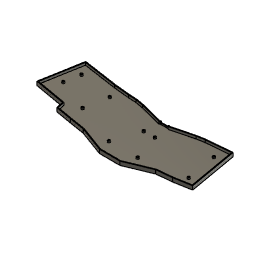
quetzal - minimal - lowpro (Autodesk Fusion 360 design; units mm, degrees)
Autodesk Fusion 360 part; units mm, degrees
note: some values were not read from the file. Set by a fixed rule: which sketch regions a step uses.
(part 1 of 15)
sketch "atreuskeypad-Edge_Cuts" plane through (0, 0, 0) normal (0, 1, 0) x (1, 0, 0)
  line L0 (156.651, -54.9359) -> (156.645, -54.9431)
  line L1 (156.607, -54.9484) -> (101.099, -40.5089)
  line L2 (25.155, -32.2997) -> (25.1539, -32.2991)
  line L3 (156.645, -54.9431) -> (156.635, -54.9446)
  line L4 (63.165, -36.1397) -> (25.155, -32.2997)
  line L5 (177.784, -54.9772) -> (177.776, -54.9799)
  line L6 (176.132, -52.9608) -> (176.134, -52.9601)
  line L7 (329.099, -144.851) -> (329.095, -144.87)
  line L8 (176.165, -52.9746) -> (176.166, -52.9765)
  line L9 (329.091, -144.889) -> (329.091, -144.889)
  line L10 (156.602, -54.8436) -> (158.121, -52.9883)
  line L11 (158.14, -52.9782) -> (158.155, -52.9702)
  line L12 (309.232, -32.2617) -> (309.24, -32.2769)
  line L13 (329.091, -144.889) -> (329.076, -144.898)
  line L14 (252.021, -37.1608) -> (252.024, -37.1613)
  line L15 (309.23, -32.261) -> (309.232, -32.2617)
  line L16 (63.1661, -36.1394) -> (63.165, -36.1397)
  line L17 (158.158, -52.971) -> (158.16, -52.97)
  line L18 (82.3387, -37.1108) -> (101.119, -40.4108)
  line L19 (177.766, -54.9747) -> (177.755, -54.9731)
  line L20 (25.1526, -32.2995) -> (-56.8492, -20.0866)
  line L21 (63.1672, -36.1399) -> (63.1661, -36.1394)
  line L22 (158.121, -52.9883) -> (158.124, -52.9871)
  line L23 (25.1539, -32.2991) -> (25.1526, -32.2995)
  line L24 (158.155, -52.9702) -> (158.158, -52.971)
  line L25 (329.091, -144.889) -> (329.091, -144.889)
  line L26 (309.212, -32.2553) -> (309.229, -32.259)
  line L27 (309.249, -32.2913) -> (329.099, -144.851)
  line L28 (233.247, -40.4916) -> (233.25, -40.4919)
  line L29 (329.099, -144.851) -> (329.099, -144.851)
  line L30 (158.124, -52.9871) -> (158.125, -52.9847)
  line L31 (176.168, -52.9774) -> (177.798, -54.8738)
  line L32 (177.798, -54.8738) -> (233.247, -40.4916)
  line L33 (-73.4847, -113.859) -> (-73.501, -113.849)
  line L34 (309.196, -32.2502) -> (309.212, -32.2553)
  line L35 (63.1739, -36.0401) -> (82.3328, -37.1101)
  line L36 (309.24, -32.2769) -> (309.249, -32.2913)
  line L37 (176.107, -53.06) -> (158.184, -53.07)
  line L38 (158.16, -52.97) -> (176.13, -52.96)
  line L39 (101.099, -40.5089) -> (82.3243, -37.2098)
  line L40 (177.755, -54.9731) -> (177.75, -54.9664)
  line L41 (329.095, -144.87) -> (329.091, -144.889)
  line L42 (158.184, -53.07) -> (156.659, -54.9317)
  line L43 (156.625, -54.9498) -> (156.616, -54.9471)
  line L44 (82.3356, -37.1114) -> (82.3387, -37.1108)
  line L45 (177.793, -54.9784) -> (177.784, -54.9772)
  line L46 (176.149, -52.968) -> (176.165, -52.9746)
  line L47 (252.024, -37.1613) -> (252.026, -37.1602)
  line L48 (233.25, -40.4919) -> (233.251, -40.4908)
  line L49 (82.3328, -37.1101) -> (82.3356, -37.1114)
  line L50 (156.659, -54.9317) -> (156.651, -54.9359)
  line L51 (156.616, -54.9471) -> (156.607, -54.9484)
  line L52 (176.134, -52.9601) -> (176.149, -52.968)
  line L53 (177.742, -54.9626) -> (176.107, -53.06)
  line L54 (177.75, -54.9664) -> (177.742, -54.9626)
  line L55 (176.166, -52.9765) -> (176.168, -52.9774)
  line L56 (82.3243, -37.2098) -> (63.1672, -36.1399)
  line L57 (177.776, -54.9799) -> (177.766, -54.9747)
  line L58 (-56.8492, -20.0866) -> (-73.4021, -113.779)
  line L59 (156.635, -54.9446) -> (156.625, -54.9498)
  line L60 (101.12, -40.4119) -> (101.123, -40.4116)
  line L61 (176.13, -52.96) -> (176.132, -52.9608)
  line L62 (101.119, -40.4108) -> (101.12, -40.4119)
  line L63 (233.251, -40.4908) -> (252.021, -37.1608)
  line L64 (158.125, -52.9847) -> (158.14, -52.9782)
  line L65 (25.1662, -32.2004) -> (63.1739, -36.0401)
  line L66 (101.123, -40.4116) -> (156.602, -54.8436)
  line L67 (309.229, -32.259) -> (309.23, -32.261)
  line L68 (252.026, -37.1602) -> (309.196, -32.2502)
  line L69 (329.099, -144.851) -> (329.099, -144.851)
  line L70 (191.739, -180.826) -> (191.729, -180.826)
  line L71 (-73.501, -113.849) -> (-73.501, -113.849)
  line L72 (5.3213, -144.859) -> (5.3127, -144.854)
  line L73 (80.4872, -157.589) -> (42.832, -151.479)
  line L74 (142.913, -180.577) -> (80.4872, -157.589)
  line L75 (291.525, -151.51) -> (253.532, -155.399)
  line L76 (5.3027, -144.852) -> (5.2973, -144.844)
  line L77 (-56.9191, -19.9896) -> (-56.9187, -19.989)
  line L78 (1.611, -127.061) -> (1.6132, -127.071)
  line L79 (-56.9293, -20.0057) -> (-56.9198, -19.9898)
  line L80 (1.5787, -127.041) -> (1.5873, -127.046)
  line L81 (-73.5092, -113.811) -> (-73.5092, -113.811)
  line L82 (5.3127, -144.854) -> (5.3027, -144.852)
  line L83 (5.2868, -144.829) -> (5.2811, -144.82)
  line L84 (-56.9006, -19.985) -> (-56.8826, -19.9805)
  line L85 (291.513, -151.41) -> (328.992, -144.819)
  line L86 (-56.9198, -19.9898) -> (-56.9191, -19.9896)
  line L87 (253.501, -155.304) -> (253.508, -155.304)
  line L88 (253.532, -155.399) -> (191.739, -180.826)
  line L89 (-73.5054, -113.829) -> (-73.5092, -113.811)
  line L90 (5.2973, -144.844) -> (5.289, -144.839)
  line L91 (1.5281, -127.133) -> (-73.4687, -113.869)
  line L92 (142.93, -180.58) -> (142.922, -180.577)
  line L93 (80.5123, -157.493) -> (80.5173, -157.493)
  line L94 (-73.4021, -113.779) -> (1.5787, -127.041)
  line L95 (-56.9392, -20.0213) -> (-56.9293, -20.0057)
  line L96 (1.5973, -127.048) -> (1.6028, -127.056)
  line L97 (329.059, -144.909) -> (291.529, -151.509)
  line L98 (328.992, -144.819) -> (309.159, -32.3537)
  line L99 (-73.5092, -113.811) -> (-73.5092, -113.811)
  line L100 (329.076, -144.898) -> (329.059, -144.909)
  line L101 (42.8317, -151.479) -> (42.8313, -151.479)
  line L102 (1.6028, -127.056) -> (1.611, -127.061)
  line L103 (-56.8826, -19.9805) -> (25.1662, -32.2004)
  line L104 (80.5173, -157.493) -> (142.939, -180.48)
  line L105 (191.71, -180.73) -> (253.501, -155.304)
  line L106 (291.527, -151.509) -> (291.525, -151.51)
  line L107 (5.3719, -144.767) -> (42.8483, -151.381)
  line L108 (1.6132, -127.071) -> (1.6189, -127.08)
  line L109 (142.939, -180.48) -> (191.71, -180.73)
  line L110 (1.6189, -127.08) -> (5.3719, -144.767)
  line L111 (253.508, -155.304) -> (253.515, -155.3)
  line L112 (-73.5092, -113.811) -> (-73.5092, -113.811)
  line L113 (5.2811, -144.82) -> (1.5281, -127.133)
  line L114 (5.289, -144.839) -> (5.2868, -144.829)
  line L115 (42.8483, -151.381) -> (80.508, -157.491)
  line L116 (1.5873, -127.046) -> (1.5973, -127.048)
  line L117 (-73.5092, -113.811) -> (-56.9392, -20.0213)
  line L118 (80.508, -157.491) -> (80.5123, -157.493)
  line L119 (253.515, -155.3) -> (291.513, -151.41)
  line L120 (42.832, -151.479) -> (42.8317, -151.479)
  line L121 (142.922, -180.577) -> (142.913, -180.577)
  line L122 (-73.501, -113.849) -> (-73.5054, -113.829)
  line L123 (-56.9187, -19.989) -> (-56.9006, -19.985)
  line L124 (233.271, -40.5889) -> (177.793, -54.9784)
  line L125 (329.059, -144.909) -> (329.059, -144.909)
  line L126 (191.72, -180.83) -> (142.93, -180.58)
  line L127 (42.8313, -151.479) -> (5.3213, -144.859)
  line L128 (191.729, -180.826) -> (191.72, -180.83)
  line L129 (309.159, -32.3537) -> (252.037, -37.2596)
  line L130 (-73.501, -113.849) -> (-73.501, -113.849)
  line L131 (291.529, -151.509) -> (291.527, -151.509)
  line L132 (-73.4687, -113.869) -> (-73.4847, -113.859)
  line L133 (329.059, -144.909) -> (329.059, -144.909)
  line L134 (252.037, -37.2596) -> (233.271, -40.5889)
sketch "Sketch2" plane through (0, 0, 0) normal (0, 1, 0) x (1, 0, 0)
extrude "Extrude1" add sketch "atreuskeypad-Edge_Cuts" along normal blind 3 contours L0 L1 L3 L4 L5 L19 L20 L21 L23 L37 L39 L40 L42 L43 L45 L50 L51 L53 L54 L56 L57 L58 L59 L78 L80 L85 L87 L93 L94 L96 L98 L102 L104 L105 L107 L108 L109 L110 L111 L115 L116 L118 L119 L124 L129 L134
sketch "atreuskeypad-F_Mask" plane through (0, 0, 0) normal (0, 1, 0) x (1, 0, 0)
  line L0 (199.475, -99.2993) -> (199.496, -99.1151)
  line L1 (132.979, -99.2592) -> (133, -99.075)
  line L2 (200.247, -98.3794) -> (200.432, -98.3626)
  line L3 (316.576, -97.7949) -> (316.753, -97.8497)
  line L4 (55.7718, -103.478) -> (55.5955, -103.42)
  line L5 (297.244, -102.904) -> (297.082, -102.814)
  line L6 (37.6083, -101.631) -> (37.6619, -101.809)
  line L7 (298.401, -102.581) -> (298.28, -102.721)
  line L8 (297.605, -102.983) -> (297.42, -102.961)
  line L9 (298.492, -102.42) -> (298.401, -102.581)
  line L10 (56.1408, -103.485) -> (55.9559, -103.5)
  line L11 (55.6199, -101.669) -> (55.7978, -101.617)
  line L12 (296.751, -101.659) -> (296.841, -101.497)
  line L13 (297.082, -102.814) -> (296.941, -102.693)
  line L14 (297.968, -102.919) -> (297.789, -102.969)
  line L15 (296.69, -102.205) -> (296.675, -102.02)
  line L16 (296.675, -102.02) -> (296.695, -101.836)
  line L17 (37.2613, -101.206) -> (37.4041, -101.324)
  line L18 (296.96, -101.355) -> (297.104, -101.239)
  line L19 (287.81, -102.867) -> (287.987, -102.922)
  line L20 (40.0114, -103.894) -> (39.8851, -103.641)
  line L21 (288.15, -103.01) -> (288.293, -103.128)
  line L22 (43.6913, -103.281) -> (43.6146, -103.553)
  line L23 (40.3638, -104.333) -> (40.172, -104.126)
  line L24 (39.9368, -101.996) -> (40.0787, -101.751)
  line L25 (288.497, -103.436) -> (288.551, -103.613)
  line L26 (39.8851, -103.641) -> (39.7957, -103.373)
  line L27 (40.0787, -101.751) -> (40.2536, -101.529)
  line L28 (288.293, -103.128) -> (288.41, -103.272)
  line L29 (39.7449, -103.095) -> (39.7338, -102.813)
  line L30 (43.1691, -104.267) -> (42.9587, -104.456)
  line L31 (41.2051, -100.946) -> (41.4822, -100.891)
  line L32 (43.3509, -104.051) -> (43.1691, -104.267)
  line L33 (42.4691, -104.735) -> (42.1997, -104.82)
  line L34 (288.487, -104.184) -> (288.395, -104.345)
  line L35 (40.9386, -101.04) -> (41.2051, -100.946)
  line L36 (40.5828, -104.512) -> (40.3638, -104.333)
  line L37 (39.7338, -102.813) -> (39.7626, -102.532)
  line L38 (43.6146, -103.553) -> (43.5004, -103.811)
  line L39 (43.5004, -103.811) -> (43.3509, -104.051)
  line L40 (42.1997, -104.82) -> (41.9211, -104.867)
  line L41 (42.8309, -101.204) -> (43.0555, -101.375)
  line L42 (39.8307, -102.257) -> (39.9368, -101.996)
  line L43 (41.085, -104.768) -> (40.8249, -104.658)
  line L44 (42.7238, -104.613) -> (42.4691, -104.735)
  line L45 (41.9211, -104.867) -> (41.6386, -104.873)
  line L46 (42.0457, -100.9) -> (42.3209, -100.964)
  line L47 (109.245, -73.0347) -> (109.335, -72.8722)
  line L48 (-35.0955, -72.3151) -> (-35.1722, -72.587)
  line L49 (-35.0539, -71.9095) -> (-35.0579, -72.0351)
  line L50 (-35.2311, -71.0865) -> (-35.1333, -71.3515)
  line L51 (215.619, -98.2785) -> (215.409, -98.467)
  line L52 (1.4974, -97.4895) -> (1.6419, -97.3733)
  line L53 (215.409, -98.467) -> (215.174, -98.624)
  line L54 (-35.6177, -73.3013) -> (-35.8281, -73.4898)
  line L55 (316.916, -97.9379) -> (317.059, -98.0561)
  line L56 (133.725, -100.2) -> (133.549, -100.143)
  line L57 (133.549, -100.143) -> (133.387, -100.053)
  line L58 (-35.7313, -70.4093) -> (-35.5331, -70.6106)
  line L59 (133.264, -98.5938) -> (133.409, -98.4776)
  line L60 (133.751, -98.3393) -> (133.936, -98.3225)
  line L61 (317.176, -98.1997) -> (317.263, -98.3634)
  line L62 (133.409, -98.4776) -> (133.573, -98.3917)
  line L63 (316.753, -97.8497) -> (316.916, -97.9379)
  line L64 (133.936, -98.3225) -> (134.12, -98.3419)
  line L65 (133, -99.075) -> (133.056, -98.8983)
  line L66 (1.6419, -97.3733) -> (1.8062, -97.2874)
  line L67 (2.1687, -97.2182) -> (2.3531, -97.2376)
  line L68 (-35.4359, -73.0851) -> (-35.6177, -73.3013)
  line L69 (200.432, -98.3626) -> (200.616, -98.382)
  line L70 (134.879, -99.2725) -> (134.879, -99.299)
  line L71 (134.861, -99.088) -> (134.879, -99.2725)
  line L72 (200.769, -100.198) -> (200.59, -100.248)
  line L73 (200.045, -100.183) -> (199.883, -100.093)
  line L74 (200.59, -100.248) -> (200.405, -100.262)
  line L75 (216.142, -97.2923) -> (216.065, -97.5642)
  line L76 (212.195, -97.1062) -> (212.184, -96.8239)
  line L77 (212.908, -95.3457) -> (213.138, -95.1814)
  line L78 (212.387, -96.0068) -> (212.529, -95.7625)
  line L79 (212.335, -97.6521) -> (212.246, -97.3841)
  line L80 (212.622, -98.1372) -> (212.462, -97.9048)
  line L81 (215.281, -95.2151) -> (215.506, -95.3865)
  line L82 (121.692, -95.5477) -> (121.86, -95.775)
  line L83 (122.092, -96.2887) -> (122.151, -96.5648)
  line L84 (119.524, -98.7388) -> (119.263, -98.6287)
  line L85 (213.655, -94.9576) -> (213.932, -94.9025)
  line L86 (214.215, -94.887) -> (214.496, -94.9113)
  line L87 (214.089, -98.8845) -> (213.808, -98.8513)
  line L88 (212.814, -98.3446) -> (212.622, -98.1372)
  line L89 (213.138, -95.1814) -> (213.389, -95.0512)
  line L90 (216.183, -96.8867) -> (216.179, -97.0123)
  line L91 (120.484, -94.8713) -> (120.759, -94.9351)
  line L92 (1.9841, -97.235) -> (2.1687, -97.2182)
  line L93 (215.801, -98.0623) -> (215.619, -98.2785)
  line L94 (216.006, -96.0637) -> (216.104, -96.3287)
  line L95 (213.535, -98.7789) -> (213.275, -98.6687)
  line L96 (121.789, -98.0222) -> (121.608, -98.2385)
  line L97 (215.174, -98.624) -> (214.919, -98.7463)
  line L98 (212.529, -95.7625) -> (212.704, -95.5407)
  line L99 (122.053, -97.5241) -> (121.939, -97.7825)
  line L100 (118.45, -97.8647) -> (118.324, -97.612)
  line L101 (215.506, -95.3865) -> (215.704, -95.5878)
  line L102 (118.269, -96.2286) -> (118.375, -95.9668)
  line L103 (118.375, -95.9668) -> (118.517, -95.7225)
  line L104 (212.246, -97.3841) -> (212.195, -97.1062)
  line L105 (121.269, -95.175) -> (121.494, -95.3464)
  line L106 (212.281, -96.2687) -> (212.387, -96.0068)
  line L107 (119.126, -95.1414) -> (119.377, -95.0111)
  line L108 (213.808, -98.8513) -> (213.535, -98.7789)
  line L109 (118.517, -95.7225) -> (118.692, -95.5006)
  line L110 (119.377, -95.0111) -> (119.644, -94.9175)
  line L111 (216.104, -96.3287) -> (216.163, -96.6049)
  line L112 (213.275, -98.6687) -> (213.033, -98.523)
  line L113 (121.494, -95.3464) -> (121.692, -95.5477)
  line L114 (122.171, -96.8466) -> (122.167, -96.9722)
  line L115 (214.65, -98.8314) -> (214.371, -98.8778)
  line L116 (121.86, -95.775) -> (121.994, -96.0236)
  line L117 (214.771, -94.9751) -> (215.035, -95.0771)
  line L118 (216.163, -96.6049) -> (216.183, -96.8867)
  line L119 (120.759, -94.9351) -> (121.023, -95.037)
  line L120 (214.371, -98.8778) -> (214.089, -98.8845)
  line L121 (214.919, -98.7463) -> (214.65, -98.8314)
  line L122 (213.932, -94.9025) -> (214.215, -94.887)
  line L123 (215.035, -95.0771) -> (215.281, -95.2151)
  line L124 (121.994, -96.0236) -> (122.092, -96.2887)
  line L125 (212.213, -96.5429) -> (212.281, -96.2687)
  line L126 (213.033, -98.523) -> (212.814, -98.3446)
  line L127 (212.184, -96.8239) -> (212.213, -96.5429)
  line L128 (1.3782, -97.6315) -> (1.4974, -97.4895)
  line L129 (212.462, -97.9048) -> (212.335, -97.6521)
  line L130 (122.151, -96.5648) -> (122.171, -96.8466)
  line L131 (213.389, -95.0512) -> (213.655, -94.9576)
  line L132 (212.704, -95.5407) -> (212.908, -95.3457)
  line L133 (121.023, -95.037) -> (121.269, -95.175)
  line L134 (215.951, -97.8226) -> (215.801, -98.0623)
  line L135 (109.235, -73.7586) -> (109.184, -73.5804)
  line L136 (-35.5331, -70.6106) -> (-35.3653, -70.8378)
  line L137 (109.169, -73.3957) -> (109.189, -73.2114)
  line L138 (134.879, -99.299) -> (134.856, -99.483)
  line L139 (201.202, -99.8602) -> (201.08, -100.001)
  line L140 (199.627, -99.8272) -> (199.542, -99.6623)
  line L141 (199.542, -99.6623) -> (199.491, -99.4841)
  line L142 (200.934, -100.115) -> (200.769, -100.198)
  line L143 (199.761, -98.6338) -> (199.905, -98.5176)
  line L144 (201.08, -100.001) -> (200.934, -100.115)
  line L145 (200.221, -100.24) -> (200.045, -100.183)
  line L146 (201.293, -99.699) -> (201.202, -99.8602)
  line L147 (198.067, -80.5785) -> (198.044, -80.7625)
  line L148 (31.1051, -80.7559) -> (31.2897, -80.7391)
  line L149 (109.454, -72.7302) -> (109.598, -72.614)
  line L150 (-35.9559, -70.2379) -> (-35.7313, -70.4093)
  line L151 (109.189, -73.2114) -> (109.245, -73.0347)
  line L152 (-35.0739, -71.6277) -> (-35.0539, -71.9095)
  line L153 (-35.8281, -73.4898) -> (-36.063, -73.6468)
  line L154 (35.8008, -101.796) -> (35.8569, -101.619)
  line L155 (35.8569, -101.619) -> (35.9462, -101.457)
  line L156 (35.9462, -101.457) -> (36.0653, -101.315)
  line L157 (35.7956, -102.165) -> (35.7801, -101.98)
  line L158 (36.0653, -101.315) -> (36.2098, -101.198)
  line L159 (36.2098, -101.198) -> (36.3742, -101.113)
  line L160 (36.3742, -101.113) -> (36.552, -101.06)
  line L161 (36.7367, -101.043) -> (36.9211, -101.063)
  line L162 (36.552, -101.06) -> (36.7367, -101.043)
  line L163 (195.735, -98.2193) -> (196.011, -98.2831)
  line L164 (36.1879, -102.773) -> (36.0467, -102.653)
  line L165 (189.485, -101.248) -> (189.47, -101.064)
  line L166 (189.736, -101.737) -> (189.621, -101.591)
  line L167 (190.426, -100.127) -> (190.611, -100.146)
  line L168 (189.899, -100.282) -> (190.064, -100.196)
  line L169 (144.126, -100.106) -> (144.303, -100.161)
  line L170 (189.47, -101.064) -> (189.49, -100.879)
  line L171 (144.867, -100.852) -> (144.885, -101.037)
  line L172 (191.369, -101.103) -> (191.346, -101.287)
  line L173 (191.075, -101.765) -> (190.929, -101.879)
  line L174 (189.636, -100.54) -> (189.755, -100.398)
  line L175 (191.288, -101.463) -> (191.196, -101.624)
  line L176 (189.878, -101.857) -> (189.736, -101.737)
  line L177 (190.039, -101.947) -> (189.878, -101.857)
  line L178 (191.346, -101.287) -> (191.288, -101.463)
  line L179 (190.585, -102.012) -> (190.4, -102.027)
  line L180 (190.216, -102.005) -> (190.039, -101.947)
  line L181 (313.071, -98.5359) -> (313.205, -98.7846)
  line L182 (309.412, -99.2637) -> (309.48, -98.9896)
  line L183 (311.695, -97.6322) -> (311.97, -97.696)
  line L184 (143.415, -100.242) -> (143.579, -100.156)
  line L185 (143.393, -101.817) -> (143.251, -101.697)
  line L186 (144.278, -101.922) -> (144.1, -101.972)
  line L187 (143.27, -100.358) -> (143.415, -100.242)
  line L188 (144.1, -101.972) -> (143.915, -101.987)
  line L189 (311.849, -101.552) -> (311.57, -101.599)
  line L190 (144.884, -101.063) -> (144.861, -101.247)
  line L191 (310.013, -101.066) -> (309.821, -100.858)
  line L192 (143.052, -101.386) -> (143, -101.208)
  line L193 (312.373, -101.345) -> (312.118, -101.467)
  line L194 (309.48, -98.9896) -> (309.586, -98.7277)
  line L195 (144.803, -101.423) -> (144.711, -101.584)
  line L196 (313.205, -98.7846) -> (313.303, -99.0496)
  line L197 (313.264, -100.285) -> (313.15, -100.543)
  line L198 (143, -101.208) -> (142.985, -101.024)
  line L199 (312.234, -97.7979) -> (312.48, -97.936)
  line L200 (312.48, -97.936) -> (312.705, -98.1074)
  line L201 (312.818, -100.999) -> (312.608, -101.188)
  line L202 (311.007, -101.572) -> (310.734, -101.5)
  line L203 (313.378, -99.7332) -> (313.341, -100.013)
  line L204 (309.383, -99.5448) -> (309.412, -99.2637)
  line L205 (144.444, -101.839) -> (144.278, -101.922)
  line L206 (309.534, -100.373) -> (309.445, -100.105)
  line L207 (312.608, -101.188) -> (312.373, -101.345)
  line L208 (313.15, -100.543) -> (313, -100.783)
  line L209 (143.731, -101.965) -> (143.554, -101.907)
  line L210 (313.341, -100.013) -> (313.264, -100.285)
  line L211 (144.711, -101.584) -> (144.59, -101.725)
  line L212 (312.705, -98.1074) -> (312.903, -98.3087)
  line L213 (144.885, -101.037) -> (144.884, -101.063)
  line L214 (143.251, -101.697) -> (143.136, -101.551)
  line L215 (310.734, -101.5) -> (310.474, -101.39)
  line L216 (144.861, -101.247) -> (144.803, -101.423)
  line L217 (142.985, -101.024) -> (143.006, -100.839)
  line L218 (313.303, -99.0496) -> (313.362, -99.3258)
  line L219 (309.586, -98.7277) -> (309.728, -98.4834)
  line L220 (189.49, -100.879) -> (189.547, -100.703)
  line L221 (189.755, -100.398) -> (189.899, -100.282)
  line L222 (143.915, -101.987) -> (143.731, -101.965)
  line L223 (143.554, -101.907) -> (143.393, -101.817)
  line L224 (311.97, -97.696) -> (312.234, -97.7979)
  line L225 (311.57, -101.599) -> (311.288, -101.605)
  line L226 (143.006, -100.839) -> (143.062, -100.663)
  line L227 (144.59, -101.725) -> (144.444, -101.839)
  line L228 (143.136, -101.551) -> (143.052, -101.386)
  line L229 (143.062, -100.663) -> (143.151, -100.5)
  line L230 (309.394, -99.8271) -> (309.383, -99.5448)
  line L231 (313.382, -99.6076) -> (313.378, -99.7332)
  line L232 (310.474, -101.39) -> (310.232, -101.244)
  line L233 (313.362, -99.3258) -> (313.382, -99.6076)
  line L234 (313, -100.783) -> (312.818, -100.999)
  line L235 (312.903, -98.3087) -> (313.071, -98.5359)
  line L236 (309.728, -98.4834) -> (309.903, -98.2616)
  line L237 (312.118, -101.467) -> (311.849, -101.552)
  line L238 (309.661, -100.626) -> (309.534, -100.373)
  line L239 (190.064, -100.196) -> (190.242, -100.144)
  line L240 (143.151, -100.5) -> (143.27, -100.358)
  line L241 (143.757, -100.104) -> (143.941, -100.087)
  line L242 (143.579, -100.156) -> (143.757, -100.104)
  line L243 (143.941, -100.087) -> (144.126, -100.106)
  line L244 (309.445, -100.105) -> (309.394, -99.8271)
  line L245 (310.337, -97.9023) -> (310.588, -97.7721)
  line L246 (21.6032, -101.025) -> (21.4114, -100.818)
  line L247 (21.4114, -100.818) -> (21.2508, -100.586)
  line L248 (21.9273, -97.8622) -> (22.178, -97.732)
  line L249 (24.9683, -99.6931) -> (24.9307, -99.9731)
  line L250 (22.3244, -101.46) -> (22.0643, -101.35)
  line L251 (307.258, -100.128) -> (307.311, -100.305)
  line L252 (22.8781, -101.565) -> (22.5975, -101.532)
  line L253 (21.8223, -101.204) -> (21.6032, -101.025)
  line L254 (24.7398, -100.503) -> (24.5903, -100.743)
  line L255 (21.493, -98.2215) -> (21.6974, -98.0265)
  line L256 (21.2508, -100.586) -> (21.1245, -100.333)
  line L257 (24.9307, -99.9731) -> (24.854, -100.245)
  line L258 (21.0702, -98.9495) -> (21.1762, -98.6876)
  line L259 (22.0643, -101.35) -> (21.8223, -101.204)
  line L260 (21.1762, -98.6876) -> (21.3181, -98.4434)
  line L261 (307.171, -99.964) -> (307.258, -100.128)
  line L262 (307.156, -101.037) -> (307.035, -101.178)
  line L263 (22.178, -97.732) -> (22.4445, -97.6384)
  line L264 (21.002, -99.2237) -> (21.0702, -98.9495)
  line L265 (20.9843, -99.787) -> (20.9733, -99.5047)
  line L266 (307.247, -100.876) -> (307.156, -101.037)
  line L267 (307.054, -99.8203) -> (307.171, -99.964)
  line L268 (24.854, -100.245) -> (24.7398, -100.503)
  line L269 (306.748, -99.614) -> (306.911, -99.7021)
  line L270 (23.5603, -97.6559) -> (23.8238, -97.7579)
  line L271 (24.0703, -97.8959) -> (24.2949, -98.0673)
  line L272 (21.1245, -100.333) -> (21.0351, -100.065)
  line L273 (310.854, -97.6785) -> (311.132, -97.6234)
  line L274 (24.8929, -99.0095) -> (24.9523, -99.2857)
  line L275 (311.414, -97.6078) -> (311.695, -97.6322)
  line L276 (310.232, -101.244) -> (310.013, -101.066)
  line L277 (311.288, -101.605) -> (311.007, -101.572)
  line L278 (24.5903, -100.743) -> (24.4085, -100.959)
  line L279 (306.911, -99.7021) -> (307.054, -99.8203)
  line L280 (20.9733, -99.5047) -> (21.002, -99.2237)
  line L281 (23.0037, -97.5678) -> (23.2851, -97.5921)
  line L282 (310.588, -97.7721) -> (310.854, -97.6785)
  line L283 (23.7085, -101.427) -> (23.4392, -101.512)
  line L284 (310.107, -98.0666) -> (310.337, -97.9023)
  line L285 (24.9523, -99.2857) -> (24.9723, -99.5675)
  line L286 (24.4931, -98.2686) -> (24.6609, -98.4959)
  line L287 (21.3181, -98.4434) -> (21.493, -98.2215)
  line L288 (21.6974, -98.0265) -> (21.9273, -97.8622)
  line L289 (21.0351, -100.065) -> (20.9843, -99.787)
  line L290 (24.2949, -98.0673) -> (24.4931, -98.2686)
  line L291 (24.6609, -98.4959) -> (24.7951, -98.7445)
  line L292 (311.132, -97.6234) -> (311.414, -97.6078)
  line L293 (23.4392, -101.512) -> (23.1605, -101.559)
  line L294 (23.1605, -101.559) -> (22.8781, -101.565)
  line L295 (24.9723, -99.5675) -> (24.9683, -99.6931)
  line L296 (23.9632, -101.305) -> (23.7085, -101.427)
  line L297 (309.821, -100.858) -> (309.661, -100.626)
  line L298 (22.4445, -97.6384) -> (22.7216, -97.5833)
  line L299 (22.7216, -97.5833) -> (23.0037, -97.5678)
  line L300 (306.57, -99.5591) -> (306.748, -99.614)
  line L301 (307.329, -100.516) -> (307.306, -100.7)
  line L302 (309.903, -98.2616) -> (310.107, -98.0666)
  line L303 (22.5975, -101.532) -> (22.3244, -101.46)
  line L304 (23.8238, -97.7579) -> (24.0703, -97.8959)
  line L305 (24.4085, -100.959) -> (24.1981, -101.148)
  line L306 (23.2851, -97.5921) -> (23.5603, -97.6559)
  line L307 (24.7951, -98.7445) -> (24.8929, -99.0095)
  line L308 (24.1981, -101.148) -> (23.9632, -101.305)
  line L309 (307.035, -101.178) -> (306.888, -101.292)
  line L310 (306.201, -99.5566) -> (306.386, -99.5397)
  line L311 (28.907, -100.265) -> (28.9251, -100.45)
  line L312 (27.9552, -101.399) -> (27.7711, -101.377)
  line L313 (305.999, -101.36) -> (305.837, -101.27)
  line L314 (27.9817, -99.4997) -> (28.1661, -99.5191)
  line L315 (305.837, -101.27) -> (305.696, -101.15)
  line L316 (305.859, -99.6948) -> (306.024, -99.6089)
  line L317 (201.375, -99.3391) -> (201.352, -99.523)
  line L318 (28.9251, -100.45) -> (28.9247, -100.476)
  line L319 (27.0252, -100.436) -> (27.0458, -100.252)
  line L320 (28.4841, -101.252) -> (28.3186, -101.335)
  line L321 (28.3432, -99.5739) -> (28.5063, -99.6621)
  line L322 (200.793, -98.4368) -> (200.957, -98.525)
  line L323 (307.311, -100.305) -> (307.329, -100.49)
  line L324 (27.1912, -99.9129) -> (27.3104, -99.7709)
  line L325 (28.843, -100.836) -> (28.7514, -100.997)
  line L326 (201.099, -98.6432) -> (201.217, -98.7869)
  line L327 (306.723, -101.375) -> (306.544, -101.425)
  line L328 (306.888, -101.292) -> (306.723, -101.375)
  line L329 (28.7664, -99.9239) -> (28.8534, -100.088)
  line L330 (201.217, -98.7869) -> (201.304, -98.9506)
  line L331 (201.357, -99.1281) -> (201.375, -99.3126)
  line L332 (306.024, -99.6089) -> (306.201, -99.5566)
  line L333 (201.375, -99.3126) -> (201.375, -99.3391)
  line L334 (305.45, -100.292) -> (305.506, -100.115)
  line L335 (306.175, -101.418) -> (305.999, -101.36)
  line L336 (305.596, -99.953) -> (305.715, -99.811)
  line L337 (27.4329, -101.23) -> (27.2917, -101.11)
  line L338 (27.0407, -100.621) -> (27.0252, -100.436)
  line L339 (28.3186, -101.335) -> (28.1401, -101.385)
  line L340 (27.7711, -101.377) -> (27.5948, -101.32)
  line L341 (307.329, -100.49) -> (307.329, -100.516)
  line L342 (305.496, -100.839) -> (305.445, -100.661)
  line L343 (201.304, -98.9506) -> (201.357, -99.1281)
  line L344 (28.6492, -99.7803) -> (28.7664, -99.9239)
  line L345 (306.544, -101.425) -> (306.36, -101.44)
  line L346 (27.2917, -101.11) -> (27.1765, -100.964)
  line L347 (27.3104, -99.7709) -> (27.4549, -99.6547)
  line L348 (201.352, -99.523) -> (201.293, -99.699)
  line L349 (27.0918, -100.799) -> (27.0407, -100.621)
  line L350 (306.386, -99.5397) -> (306.57, -99.5591)
  line L351 (305.581, -101.004) -> (305.496, -100.839)
  line L352 (28.8534, -100.088) -> (28.907, -100.265)
  line L353 (305.715, -99.811) -> (305.859, -99.6948)
  line L354 (28.9247, -100.476) -> (28.9015, -100.66)
  line L355 (28.9015, -100.66) -> (28.843, -100.836)
  line L356 (28.1661, -99.5191) -> (28.3432, -99.5739)
  line L357 (306.36, -101.44) -> (306.175, -101.418)
  line L358 (305.445, -100.661) -> (305.43, -100.476)
  line L359 (305.506, -100.115) -> (305.596, -99.953)
  line L360 (27.1765, -100.964) -> (27.0918, -100.799)
  line L361 (305.696, -101.15) -> (305.581, -101.004)
  line L362 (28.5063, -99.6621) -> (28.6492, -99.7803)
  line L363 (28.1401, -101.385) -> (27.9552, -101.399)
  line L364 (27.7971, -99.5165) -> (27.9817, -99.4997)
  line L365 (305.43, -100.476) -> (305.45, -100.292)
  line L366 (27.5948, -101.32) -> (27.4329, -101.23)
  line L367 (307.306, -100.7) -> (307.247, -100.876)
  line L368 (200.957, -98.525) -> (201.099, -98.6432)
  line L369 (28.7514, -100.997) -> (28.6302, -101.138)
  line L370 (28.6302, -101.138) -> (28.4841, -101.252)
  line L371 (27.0458, -100.252) -> (27.1019, -100.075)
  line L372 (27.6192, -99.5688) -> (27.7971, -99.5165)
  line L373 (27.1019, -100.075) -> (27.1912, -99.9129)
  line L374 (27.4549, -99.6547) -> (27.6192, -99.5688)
  line L375 (200.616, -98.382) -> (200.793, -98.4368)
  line L376 (199.552, -98.9383) -> (199.641, -98.7759)
  line L377 (199.641, -98.7759) -> (199.761, -98.6338)
  line L378 (134.12, -98.3419) -> (134.297, -98.3967)
  line L379 (200.069, -98.4317) -> (200.247, -98.3794)
  line L380 (199.905, -98.5176) -> (200.069, -98.4317)
  line L381 (199.883, -100.093) -> (199.742, -99.9725)
  line L382 (199.742, -99.9725) -> (199.627, -99.8272)
  line L383 (199.491, -99.4841) -> (199.475, -99.2993)
  line L384 (134.603, -98.6031) -> (134.72, -98.7468)
  line L385 (134.46, -98.4849) -> (134.603, -98.6031)
  line L386 (199.496, -99.1151) -> (199.552, -98.9383)
  line L387 (134.807, -98.9105) -> (134.861, -99.088)
  line L388 (134.72, -98.7468) -> (134.807, -98.9105)
  line L389 (200.405, -100.262) -> (200.221, -100.24)
  line L390 (134.297, -98.3967) -> (134.46, -98.4849)
  line L391 (191.196, -101.624) -> (191.075, -101.765)
  line L392 (190.4, -102.027) -> (190.216, -102.005)
  line L393 (144.609, -100.367) -> (144.726, -100.511)
  line L394 (190.242, -100.144) -> (190.426, -100.127)
  line L395 (144.726, -100.511) -> (144.813, -100.675)
  line L396 (144.303, -100.161) -> (144.466, -100.249)
  line L397 (144.813, -100.675) -> (144.867, -100.852)
  line L398 (190.929, -101.879) -> (190.763, -101.963)
  line L399 (189.547, -100.703) -> (189.636, -100.54)
  line L400 (189.536, -101.427) -> (189.485, -101.248)
  line L401 (190.611, -100.146) -> (190.788, -100.201)
  line L402 (191.352, -100.892) -> (191.37, -101.077)
  line L403 (138.284, -102.047) -> (138.024, -101.937)
  line L404 (138.557, -102.119) -> (138.284, -102.047)
  line L405 (137.563, -101.613) -> (137.371, -101.405)
  line L406 (136.933, -100.092) -> (136.962, -99.8108)
  line L407 (137.278, -99.0305) -> (137.453, -98.8086)
  line L408 (191.211, -100.551) -> (191.298, -100.715)
  line L409 (136.962, -99.8108) -> (137.03, -99.5366)
  line L410 (137.211, -101.173) -> (137.084, -100.92)
  line L411 (137.136, -99.2748) -> (137.278, -99.0305)
  line L412 (191.094, -100.407) -> (191.211, -100.551)
  line L413 (191.298, -100.715) -> (191.352, -100.892)
  line L414 (190.951, -100.289) -> (191.094, -100.407)
  line L415 (138.838, -102.152) -> (138.557, -102.119)
  line L416 (138.404, -98.2255) -> (138.681, -98.1704)
  line L417 (137.782, -101.791) -> (137.563, -101.613)
  line L418 (191.37, -101.077) -> (191.369, -101.103)
  line L419 (138.024, -101.937) -> (137.782, -101.791)
  line L420 (137.657, -98.6136) -> (137.887, -98.4494)
  line L421 (137.371, -101.405) -> (137.211, -101.173)
  line L422 (136.944, -100.374) -> (136.933, -100.092)
  line L423 (139.12, -102.146) -> (138.838, -102.152)
  line L424 (138.681, -98.1704) -> (138.963, -98.1549)
  line L425 (190.763, -101.963) -> (190.585, -102.012)
  line L426 (138.963, -98.1549) -> (139.245, -98.1793)
  line L427 (144.466, -100.249) -> (144.609, -100.367)
  line L428 (189.621, -101.591) -> (189.536, -101.427)
  line L429 (137.03, -99.5366) -> (137.136, -99.2748)
  line L430 (136.995, -100.652) -> (136.944, -100.374)
  line L431 (194.895, -98.2656) -> (195.172, -98.2105)
  line L432 (139.245, -98.1793) -> (139.52, -98.2431)
  line L433 (139.52, -98.2431) -> (139.784, -98.345)
  line L434 (140.255, -98.6544) -> (140.453, -98.8557)
  line L435 (190.788, -100.201) -> (190.951, -100.289)
  line L436 (137.084, -100.92) -> (136.995, -100.652)
  line L437 (138.138, -98.3191) -> (138.404, -98.2255)
  line L438 (137.453, -98.8086) -> (137.657, -98.6136)
  line L439 (137.887, -98.4494) -> (138.138, -98.3191)
  line L440 (140.158, -101.735) -> (139.923, -101.892)
  line L441 (194.628, -98.3592) -> (194.895, -98.2656)
  line L442 (140.368, -101.546) -> (140.158, -101.735)
  line L443 (140.755, -99.3316) -> (140.853, -99.5967)
  line L444 (193.943, -98.8487) -> (194.148, -98.6537)
  line L445 (193.626, -99.3148) -> (193.768, -99.0705)
  line L446 (139.923, -101.892) -> (139.668, -102.014)
  line L447 (195.454, -98.195) -> (195.735, -98.2193)
  line L448 (140.453, -98.8557) -> (140.621, -99.083)
  line L449 (195.172, -98.2105) -> (195.454, -98.195)
  line L450 (139.668, -102.014) -> (139.399, -102.099)
  line L451 (139.399, -102.099) -> (139.12, -102.146)
  line L452 (140.55, -101.33) -> (140.368, -101.546)
  line L453 (140.621, -99.083) -> (140.755, -99.3316)
  line L454 (140.7, -101.091) -> (140.55, -101.33)
  line L455 (292.371, -100.931) -> (292.653, -100.916)
  line L456 (43.7329, -102.876) -> (43.7289, -103.001)
  line L457 (41.6386, -104.873) -> (41.3581, -104.84)
  line L458 (42.3209, -100.964) -> (42.5844, -101.066)
  line L459 (40.8249, -104.658) -> (40.5828, -104.512)
  line L460 (42.9587, -104.456) -> (42.7238, -104.613)
  line L461 (43.5557, -102.052) -> (43.6534, -102.318)
  line L462 (43.6534, -102.318) -> (43.7129, -102.594)
  line L463 (42.5844, -101.066) -> (42.8309, -101.204)
  line L464 (292.653, -100.916) -> (292.935, -100.94)
  line L465 (40.172, -104.126) -> (40.0114, -103.894)
  line L466 (41.3581, -104.84) -> (41.085, -104.768)
  line L467 (43.0555, -101.375) -> (43.2537, -101.577)
  line L468 (43.2537, -101.577) -> (43.4215, -101.804)
  line L469 (43.7129, -102.594) -> (43.7329, -102.876)
  line L470 (43.4215, -101.804) -> (43.5557, -102.052)
  line L471 (43.7289, -103.001) -> (43.6913, -103.281)
  line L472 (140.912, -99.8728) -> (140.932, -100.155)
  line L473 (194.378, -98.4894) -> (194.628, -98.3592)
  line L474 (193.768, -99.0705) -> (193.943, -98.8487)
  line L475 (139.784, -98.345) -> (140.03, -98.483)
  line L476 (140.03, -98.483) -> (140.255, -98.6544)
  line L477 (140.932, -100.155) -> (140.928, -100.28)
  line L478 (140.928, -100.28) -> (140.89, -100.56)
  line L479 (140.89, -100.56) -> (140.814, -100.832)
  line L480 (140.814, -100.832) -> (140.7, -101.091)
  line L481 (194.148, -98.6537) -> (194.378, -98.4894)
  line L482 (193.52, -99.5767) -> (193.626, -99.3148)
  line L483 (140.853, -99.5967) -> (140.912, -99.8728)
  line L484 (-34.5828, -92.0998) -> (-34.704, -92.2402)
  line L485 (-34.5678, -91.0265) -> (-34.4808, -91.1902)
  line L486 (-40.8897, -88.741) -> (-40.6126, -88.6859)
  line L487 (-34.704, -92.2402) -> (-34.8501, -92.3543)
  line L488 (-41.4069, -88.9648) -> (-41.1562, -88.8346)
  line L489 (-35.1681, -90.6216) -> (-34.991, -90.6765)
  line L490 (-34.8501, -92.3543) -> (-35.0156, -92.4379)
  line L491 (-35.0156, -92.4379) -> (-35.1941, -92.4878)
  line L492 (193.452, -99.8508) -> (193.52, -99.5767)
  line L493 (-34.4912, -91.9386) -> (-34.5828, -92.0998)
  line L494 (-35.379, -92.502) -> (-35.5631, -92.4801)
  line L495 (-34.4091, -91.5522) -> (-34.4095, -91.5787)
  line L496 (-34.685, -90.8828) -> (-34.5678, -91.0265)
  line L497 (-35.7394, -92.4228) -> (-35.9013, -92.3323)
  line L498 (-41.1562, -88.8346) -> (-40.8897, -88.741)
  line L499 (-40.3305, -88.6703) -> (-40.0491, -88.6947)
  line L500 (-34.4808, -91.1902) -> (-34.4272, -91.3677)
  line L501 (-34.4327, -91.7627) -> (-34.4912, -91.9386)
  line L502 (-35.9013, -92.3323) -> (-36.0425, -92.2121)
  line L503 (-34.4095, -91.5787) -> (-34.4327, -91.7627)
  line L504 (-34.4272, -91.3677) -> (-34.4091, -91.5522)
  line L505 (-34.991, -90.6765) -> (-34.8279, -90.7646)
  line L506 (-36.0425, -92.2121) -> (-36.1576, -92.0668)
  line L507 (-36.2935, -91.7237) -> (-36.309, -91.539)
  line L508 (-36.2424, -91.9019) -> (-36.2935, -91.7237)
  line L509 (-36.1576, -92.0668) -> (-36.2424, -91.9019)
  line L510 (-36.309, -91.539) -> (-36.2884, -91.3547)
  line L511 (-36.2884, -91.3547) -> (-36.2323, -91.178)
  line L512 (-36.2323, -91.178) -> (-36.143, -91.0155)
  line L513 (-40.6126, -88.6859) -> (-40.3305, -88.6703)
  line L514 (317.059, -98.0561) -> (317.176, -98.1997)
  line L515 (133.145, -98.7358) -> (133.264, -98.5938)
  line L516 (133.131, -99.7871) -> (133.046, -99.6222)
  line L517 (-34.8279, -90.7646) -> (-34.685, -90.8828)
  line L518 (-35.5631, -92.4801) -> (-35.7394, -92.4228)
  line L519 (36.3497, -102.864) -> (36.1879, -102.773)
  line L520 (37.0736, -102.879) -> (36.895, -102.929)
  line L521 (196.011, -98.2831) -> (196.274, -98.3851)
  line L522 (37.5063, -102.541) -> (37.3852, -102.681)
  line L523 (35.9315, -102.508) -> (35.8467, -102.343)
  line L524 (35.7801, -101.98) -> (35.8008, -101.796)
  line L525 (36.0467, -102.653) -> (35.9315, -102.508)
  line L526 (-35.1941, -92.4878) -> (-35.379, -92.502)
  line L527 (296.741, -102.383) -> (296.69, -102.205)
  line L528 (298.28, -102.721) -> (298.134, -102.836)
  line L529 (297.42, -102.961) -> (297.244, -102.904)
  line L530 (297.104, -101.239) -> (297.269, -101.153)
  line L531 (296.826, -102.548) -> (296.741, -102.383)
  line L532 (297.269, -101.153) -> (297.446, -101.1)
  line L533 (37.3852, -102.681) -> (37.2391, -102.796)
  line L534 (36.7101, -102.943) -> (36.526, -102.921)
  line L535 (36.526, -102.921) -> (36.3497, -102.864)
  line L536 (37.5979, -102.38) -> (37.5063, -102.541)
  line L537 (35.8467, -102.343) -> (35.7956, -102.165)
  line L538 (36.895, -102.929) -> (36.7101, -102.943)
  line L539 (37.2391, -102.796) -> (37.0736, -102.879)
  line L540 (297.789, -102.969) -> (297.605, -102.983)
  line L541 (259.144, -124.465) -> (258.963, -124.681)
  line L542 (258.752, -124.87) -> (258.517, -125.027)
  line L543 (257.152, -125.254) -> (256.879, -125.182)
  line L544 (255.556, -122.945) -> (255.624, -122.671)
  line L545 (258.963, -124.681) -> (258.752, -124.87)
  line L546 (259.294, -124.225) -> (259.144, -124.465)
  line L547 (256.879, -125.182) -> (256.618, -125.071)
  line L548 (256.047, -121.943) -> (256.251, -121.748)
  line L549 (255.527, -123.227) -> (255.556, -122.945)
  line L550 (77.0164, -125.24) -> (76.7339, -125.247)
  line L551 (78.349, -121.95) -> (78.5168, -122.178)
  line L552 (78.8082, -122.967) -> (78.8282, -123.249)
  line L553 (255.624, -122.671) -> (255.73, -122.409)
  line L554 (78.7488, -122.691) -> (78.8082, -122.967)
  line L555 (78.4462, -124.425) -> (78.2644, -124.641)
  line L556 (259.408, -123.967) -> (259.294, -124.225)
  line L557 (256.481, -121.584) -> (256.732, -121.454)
  line L558 (259.522, -123.415) -> (259.485, -123.695)
  line L559 (258.517, -125.027) -> (258.263, -125.149)
  line L560 (258.263, -125.149) -> (257.993, -125.234)
  line L561 (255.965, -124.54) -> (255.805, -124.307)
  line L562 (255.872, -122.165) -> (256.047, -121.943)
  line L563 (256.999, -121.36) -> (257.276, -121.305)
  line L564 (256.157, -124.747) -> (255.965, -124.54)
  line L565 (256.376, -124.926) -> (256.157, -124.747)
  line L566 (255.589, -123.787) -> (255.538, -123.509)
  line L567 (256.732, -121.454) -> (256.999, -121.36)
  line L568 (259.485, -123.695) -> (259.408, -123.967)
  line L569 (256.618, -125.071) -> (256.376, -124.926)
  line L570 (257.432, -125.287) -> (257.152, -125.254)
  line L571 (255.805, -124.307) -> (255.679, -124.055)
  line L572 (255.679, -124.055) -> (255.589, -123.787)
  line L573 (76.1803, -125.141) -> (75.9202, -125.031)
  line L574 (78.1508, -121.749) -> (78.349, -121.95)
  line L575 (78.2644, -124.641) -> (78.054, -124.83)
  line L576 (75.9202, -125.031) -> (75.6782, -124.886)
  line L577 (109.431, -133.124) -> (109.485, -133.301)
  line L578 (109.084, -132.698) -> (109.227, -132.816)
  line L579 (108.896, -134.371) -> (108.718, -134.421)
  line L580 (109.42, -133.872) -> (109.329, -134.033)
  line L581 (108.533, -134.435) -> (108.349, -134.414)
  line L582 (306.725, -133.37) -> (306.477, -133.265)
  line L583 (306.347, -129.952) -> (306.585, -129.828)
  line L584 (307.637, -129.695) -> (307.899, -129.756)
  line L585 (308.596, -130.147) -> (308.785, -130.338)
  line L586 (308.944, -130.554) -> (309.072, -130.79)
  line L587 (309.201, -131.957) -> (309.128, -132.216)
  line L588 (107.679, -133.111) -> (107.769, -132.949)
  line L589 (309.221, -131.304) -> (309.24, -131.572)
  line L590 (239.751, -126.937) -> (240.014, -127.039)
  line L591 (308.039, -133.339) -> (307.784, -133.42)
  line L592 (240.261, -127.177) -> (240.485, -127.348)
  line L593 (305.468, -131.245) -> (305.533, -130.985)
  line L594 (240.986, -128.026) -> (241.083, -128.291)
  line L595 (306.247, -133.126) -> (306.039, -132.957)
  line L596 (305.441, -131.512) -> (305.468, -131.245)
  line L597 (240.851, -127.777) -> (240.986, -128.026)
  line L598 (306.477, -133.265) -> (306.247, -133.126)
  line L599 (306.585, -129.828) -> (306.839, -129.739)
  line L600 (309.128, -132.216) -> (309.019, -132.461)
  line L601 (240.684, -127.55) -> (240.851, -127.777)
  line L602 (309.072, -130.79) -> (309.165, -131.042)
  line L603 (309.24, -131.572) -> (309.236, -131.691)
  line L604 (108.375, -132.553) -> (108.559, -132.536)
  line L605 (309.019, -132.461) -> (308.877, -132.689)
  line L606 (307.784, -133.42) -> (307.519, -133.464)
  line L607 (308.383, -129.984) -> (308.596, -130.147)
  line L608 (108.559, -132.536) -> (108.744, -132.555)
  line L609 (308.505, -133.073) -> (308.281, -133.222)
  line L610 (107.618, -133.657) -> (107.603, -133.472)
  line L611 (308.785, -130.338) -> (308.944, -130.554)
  line L612 (308.704, -132.894) -> (308.505, -133.073)
  line L613 (305.585, -132.299) -> (305.5, -132.045)
  line L614 (240.014, -127.039) -> (240.261, -127.177)
  line L615 (107.769, -132.949) -> (107.888, -132.807)
  line L616 (107.603, -133.472) -> (107.623, -133.288)
  line L617 (308.281, -133.222) -> (308.039, -133.339)
  line L618 (307.519, -133.464) -> (307.25, -133.47)
  line L619 (108.197, -132.605) -> (108.375, -132.553)
  line L620 (108.032, -132.691) -> (108.197, -132.605)
  line L621 (309.236, -131.691) -> (309.201, -131.957)
  line L622 (239.476, -126.873) -> (239.751, -126.937)
  line L623 (306.984, -133.438) -> (306.725, -133.37)
  line L624 (307.25, -133.47) -> (306.984, -133.438)
  line L625 (305.634, -130.736) -> (305.769, -130.504)
  line L626 (308.877, -132.689) -> (308.704, -132.894)
  line L627 (309.165, -131.042) -> (309.221, -131.304)
  line L628 (107.623, -133.288) -> (107.679, -133.111)
  line L629 (307.899, -129.756) -> (308.149, -129.853)
  line L630 (307.37, -129.672) -> (307.637, -129.695)
  line L631 (308.149, -129.853) -> (308.383, -129.984)
  line L632 (107.888, -132.807) -> (108.032, -132.691)
  line L633 (97.1502, -129.214) -> (97.0736, -129.486)
  line L634 (305.5, -132.045) -> (305.451, -131.78)
  line L635 (237.441, -129.867) -> (237.315, -129.614)
  line L636 (237.261, -128.231) -> (237.367, -127.969)
  line L637 (97.1718, -128.527) -> (97.1918, -128.809)
  line L638 (237.315, -129.614) -> (237.226, -129.346)
  line L639 (237.509, -127.724) -> (237.683, -127.503)
  line L640 (96.5144, -127.308) -> (96.7126, -127.51)
  line L641 (95.928, -130.668) -> (95.6587, -130.753)
  line L642 (94.2838, -130.591) -> (94.0418, -130.445)
  line L643 (305.857, -132.76) -> (305.705, -132.539)
  line L644 (239.63, -130.793) -> (239.351, -130.84)
  line L645 (305.533, -130.985) -> (305.634, -130.736)
  line L646 (237.602, -130.099) -> (237.441, -129.867)
  line L647 (238.013, -130.485) -> (237.794, -130.307)
  line L648 (96.8804, -127.737) -> (97.0146, -127.986)
  line L649 (94.544, -130.701) -> (94.2838, -130.591)
  line L650 (94.0418, -130.445) -> (93.8227, -130.266)
  line L651 (305.451, -131.78) -> (305.441, -131.512)
  line L652 (238.788, -130.813) -> (238.515, -130.741)
  line L653 (238.368, -127.013) -> (238.635, -126.92)
  line L654 (97.1878, -128.934) -> (97.1502, -129.214)
  line L655 (97.1918, -128.809) -> (97.1878, -128.934)
  line L656 (237.192, -128.505) -> (237.261, -128.231)
  line L657 (240.781, -130.024) -> (240.599, -130.24)
  line L658 (95.7799, -126.897) -> (96.0433, -126.999)
  line L659 (240.389, -130.429) -> (240.154, -130.586)
  line L660 (241.121, -129.254) -> (241.044, -129.526)
  line L661 (238.255, -130.631) -> (238.013, -130.485)
  line L662 (240.485, -127.348) -> (240.684, -127.55)
  line L663 (241.083, -128.291) -> (241.143, -128.567)
  line L664 (238.912, -126.864) -> (239.194, -126.849)
  line L665 (96.0433, -126.999) -> (96.2898, -127.137)
  line L666 (95.6587, -130.753) -> (95.38, -130.8)
  line L667 (241.143, -128.567) -> (241.163, -128.849)
  line L668 (97.1124, -128.251) -> (97.1718, -128.527)
  line L669 (305.935, -130.293) -> (306.129, -130.108)
  line L670 (237.683, -127.503) -> (237.888, -127.308)
  line L671 (241.044, -129.526) -> (240.93, -129.784)
  line L672 (305.769, -130.504) -> (305.935, -130.293)
  line L673 (237.164, -128.786) -> (237.192, -128.505)
  line L674 (306.039, -132.957) -> (305.857, -132.76)
  line L675 (237.175, -129.068) -> (237.164, -128.786)
  line L676 (240.154, -130.586) -> (239.899, -130.708)
  line L677 (241.163, -128.849) -> (241.159, -128.974)
  line L678 (239.069, -130.846) -> (238.788, -130.813)
  line L679 (305.705, -132.539) -> (305.585, -132.299)
  line L680 (237.367, -127.969) -> (237.509, -127.724)
  line L681 (240.599, -130.24) -> (240.389, -130.429)
  line L682 (238.118, -127.143) -> (238.368, -127.013)
  line L683 (238.515, -130.741) -> (238.255, -130.631)
  line L684 (237.226, -129.346) -> (237.175, -129.068)
  line L685 (307.102, -129.687) -> (307.37, -129.672)
  line L686 (239.899, -130.708) -> (239.63, -130.793)
  line L687 (306.839, -129.739) -> (307.102, -129.687)
  line L688 (241.159, -128.974) -> (241.121, -129.254)
  line L689 (240.93, -129.784) -> (240.781, -130.024)
  line L690 (97.0146, -127.986) -> (97.1124, -128.251)
  line L691 (239.351, -130.84) -> (239.069, -130.846)
  line L692 (96.2898, -127.137) -> (96.5144, -127.308)
  line L693 (238.635, -126.92) -> (238.912, -126.864)
  line L694 (237.794, -130.307) -> (237.602, -130.099)
  line L695 (237.888, -127.308) -> (238.118, -127.143)
  line L696 (306.129, -130.108) -> (306.347, -129.952)
  line L697 (94.664, -126.879) -> (94.9411, -126.824)
  line L698 (234.834, -129.061) -> (234.951, -129.205)
  line L699 (235.11, -129.757) -> (235.086, -129.941)
  line L700 (96.4176, -130.389) -> (96.1827, -130.546)
  line L701 (93.1928, -128.746) -> (93.2216, -128.465)
  line L702 (101.121, -129.901) -> (101.062, -130.077)
  line L703 (94.3975, -126.973) -> (94.664, -126.879)
  line L704 (97.0736, -129.486) -> (96.9593, -129.744)
  line L705 (100.386, -128.76) -> (100.563, -128.815)
  line L706 (95.38, -130.8) -> (95.0976, -130.806)
  line L707 (233.495, -129.052) -> (233.64, -128.936)
  line L708 (234.325, -130.666) -> (234.14, -130.681)
  line L709 (100.869, -129.021) -> (100.986, -129.165)
  line L710 (233.64, -128.936) -> (233.804, -128.85)
  line L711 (95.5047, -126.833) -> (95.7799, -126.897)
  line L712 (233.804, -128.85) -> (233.982, -128.798)
  line L713 (233.376, -129.194) -> (233.495, -129.052)
  line L714 (93.6309, -130.059) -> (93.4703, -129.827)
  line L715 (93.2897, -128.191) -> (93.3957, -127.929)
  line L716 (93.7125, -127.463) -> (93.9169, -127.268)
  line L717 (96.1827, -130.546) -> (95.928, -130.668)
  line L718 (93.2216, -128.465) -> (93.2897, -128.191)
  line L719 (234.503, -130.616) -> (234.325, -130.666)
  line L720 (95.0976, -130.806) -> (94.817, -130.773)
  line L721 (235.038, -129.369) -> (235.092, -129.546)
  line L722 (100.563, -128.815) -> (100.726, -128.903)
  line L723 (93.2039, -129.028) -> (93.1928, -128.746)
  line L724 (100.986, -129.165) -> (101.073, -129.329)
  line L725 (101.062, -130.077) -> (100.971, -130.238)
  line L726 (93.2546, -129.306) -> (93.2039, -129.028)
  line L727 (100.971, -130.238) -> (100.85, -130.379)
  line L728 (234.669, -130.533) -> (234.503, -130.616)
  line L729 (233.287, -129.357) -> (233.376, -129.194)
  line L730 (235.028, -130.117) -> (234.936, -130.278)
  line L731 (234.951, -129.205) -> (235.038, -129.369)
  line L732 (100.726, -128.903) -> (100.869, -129.021)
  line L733 (100.704, -130.493) -> (100.538, -130.576)
  line L734 (93.344, -129.574) -> (93.2546, -129.306)
  line L735 (96.7126, -127.51) -> (96.8804, -127.737)
  line L736 (234.691, -128.943) -> (234.834, -129.061)
  line L737 (235.086, -129.941) -> (235.028, -130.117)
  line L738 (234.815, -130.419) -> (234.669, -130.533)
  line L739 (233.477, -130.391) -> (233.361, -130.245)
  line L740 (93.3957, -127.929) -> (93.5376, -127.684)
  line L741 (233.21, -129.717) -> (233.231, -129.533)
  line L742 (234.528, -128.855) -> (234.691, -128.943)
  line L743 (100.85, -130.379) -> (100.704, -130.493)
  line L744 (233.361, -130.245) -> (233.277, -130.08)
  line L745 (93.8227, -130.266) -> (93.6309, -130.059)
  line L746 (239.194, -126.849) -> (239.476, -126.873)
  line L747 (96.9593, -129.744) -> (96.8098, -129.984)
  line L748 (93.9169, -127.268) -> (94.1468, -127.103)
  line L749 (234.351, -128.8) -> (234.528, -128.855)
  line L750 (96.8098, -129.984) -> (96.628, -130.2)
  line L751 (95.2232, -126.809) -> (95.5047, -126.833)
  line L752 (235.11, -129.731) -> (235.11, -129.757)
  line L753 (94.9411, -126.824) -> (95.2232, -126.809)
  line L754 (96.628, -130.2) -> (96.4176, -130.389)
  line L755 (93.5376, -127.684) -> (93.7125, -127.463)
  line L756 (234.936, -130.278) -> (234.815, -130.419)
  line L757 (235.092, -129.546) -> (235.11, -129.731)
  line L758 (94.817, -130.773) -> (94.544, -130.701)
  line L759 (94.1468, -127.103) -> (94.3975, -126.973)
  line L760 (93.4703, -129.827) -> (93.344, -129.574)
  line L761 (244.697, -127.179) -> (244.84, -127.297)
  line L762 (101.144, -129.717) -> (101.121, -129.901)
  line L763 (100.175, -130.64) -> (99.9906, -130.619)
  line L764 (244.534, -127.091) -> (244.697, -127.179)
  line L765 (243.367, -128.481) -> (243.282, -128.316)
  line L766 (233.277, -130.08) -> (233.225, -129.902)
  line L767 (101.145, -129.691) -> (101.144, -129.717)